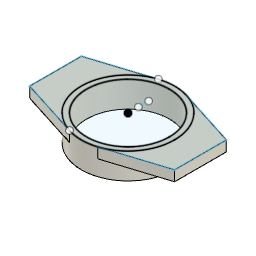
無題 (Autodesk Fusion 360 design; units mm, degrees)
Autodesk Fusion 360 part; units mm, degrees
sketch "スケッチ1" plane through (0, 0, 0) normal (0, 0, 1) x (1, 0, 0)
  circle A0 centre (0, 0) radius 10.5
  circle A1 centre (0, 0) radius 9.5
  circle A2 centre (0, 0) radius 9
  circle A3 centre (0, 0) radius 8
  dimension "d1" = 21
  dimension "d2" = 19
  dimension "d3" = 18
  dimension "d4" = 16
  constraint coincident A0.centre A1.centre
  measures "d1" diameter of A0
  measures "d2" diameter of A1
  measures "d3" diameter of A2
  measures "d4" diameter of A3
extrude "押し出し1" add sketch "スケッチ1" along normal blind 6 contours A0 makes body 1
extrude "押し出し2" add sketch "スケッチ1" along normal blind 6 separate body contours A2 makes body 2
sketch "スケッチ2" plane through (0, 0, 6) normal (0, 0, 1) x (-1, 0, 0)
  circle A0 centre (0, 0) radius 9.5
  circle A1 centre (0, 0) radius 10.5
  line L0 (2, -15) -> (-2, -15)
  line L1 (-2, -15) -> (-8.4577, -6.2223)
  line L2 (2, -15) -> (8.4577, -6.2223)
  line L3 (0, 0) -> (-3.4838, 0)
  line L4 (2, 15) -> (8.4577, 6.2223)
  line L5 (2, 15) -> (-2, 15)
  line L6 (-2, 15) -> (-8.4577, 6.2223)
  constraint horizontal L0
  constraint coincident A1 L1.end
  constraint tangent A1 L1
  constraint coincident A1 L2.end
  constraint tangent A1 L2
  constraint coincident A0.centre A1.centre
  constraint parallel L0 L3
  constraint symmetric L0.start L3 L4.start
  constraint symmetric L0.end L3 L5.end
  constraint symmetric L1.end L3 L6.end
  constraint symmetric L2.end L3 L4.end
extrude "押し出し3" add sketch "スケッチ2" against normal blind 2 contours A1 L4 L5 L6 | A1 L0 L1 L2 bodies 1
sketch "スケッチ3" plane through (0, 0, 6) normal (0, 0, 1) x (-1, 0, 0)
  circle A0 centre (0, 0) radius 8
  circle A1 centre (0, 0) radius 9
  line L0 (-15, -2) -> (-15, 2)
  line L1 (-15, 2) -> (-4.3494, 7.8792)
  line L2 (-15, 0) -> (-12.4057, 0)
  line L3 (-15, -2) -> (-4.3494, -7.8792)
  line L4 (0, 0) -> (0, -2)
  line L5 (15, -2) -> (4.3494, -7.8792)
  line L6 (15, -2) -> (15, 2)
  line L7 (15, 2) -> (4.3494, 7.8792)
  constraint vertical L0
  constraint coincident A1 L1.end
  constraint tangent A1 L1
  constraint midpoint L0 L2.start
  constraint perpendicular L0 L2
  constraint symmetric L0.end L2 L0.start
  constraint symmetric L1.end L2 L3.end
  constraint coincident A0.centre A1.centre
  constraint vertical L4
  constraint symmetric L0.start L4 L5.start
  constraint symmetric L0.end L4 L6.end
  constraint symmetric L1.end L4 L7.end
  constraint symmetric L3.end L4 L5.end
extrude "押し出し4" add sketch "スケッチ3" along normal blind 2 separate body makes body 3
combine "結合1" operation add target body 3 tool bodies 2
sketch "スケッチ1 (2)" plane through (0, 0, 0) normal (0, 0, 1) x (1, 0, 0) in component "Component'"
  circle A0 centre (0, 0) radius 11.25
  circle A1 centre (0, 0) radius 9.75
  line L0 (-2.095, 15.0718) -> (2.1708, 15.0718)
  line L1 (2.1708, 15.0718) -> (8.6891, 7.1458)
  line L2 (-2.095, 15.0718) -> (-8.6482, 7.1952)
  line L3 (-5.0595, -20.013) -> (5.0595, -20.013)
  line L4 (5.0595, -20.013) -> (10.6475, -3.6322)
  line L5 (-5.0595, -20.013) -> (-10.6475, -3.6322)
  dimension "d13" = 22.5
  dimension "d14" = 19.5
  constraint coincident A0.centre A1.centre
  constraint concentric A0 A1
  constraint horizontal L0
  constraint coincident A0 L1.end
  constraint tangent A0 L1
  constraint coincident A0 L2.end
  constraint tangent A0 L2
  constraint horizontal L3
  constraint coincident A0 L4.end
  constraint tangent A0 L4
  constraint coincident A0 L5.end
  constraint tangent A0 L5
  measures "d13" diameter of A0
  measures "d14" diameter of A1
extrude "押し出し1'" add sketch "スケッチ1 (2)" against normal blind 2 separate body makes body 4 in component "Component'"
extrude "押し出し2'" add sketch "スケッチ1 (2)" against normal blind 5 contours A0 bodies 4 in component "Component'"
sketch "スケッチ2 (2)" plane through (0, 0, 0) normal (0, 0, 1) x (1, 0, 0) in component "Component'"
  circle A0 centre (0, 0) radius 9
  circle A1 centre (0, 0) radius 8
  line L0 (14, 5) -> (14, -5)
  line L1 (14, -5) -> (2.722, -8.5785)
  line L2 (14, 5) -> (2.722, 8.5785)
  line L3 (0, 2) -> (0, 4)
  line L4 (-14, 5) -> (-14, -5)
  line L5 (-14, 5) -> (-2.722, 8.5785)
  line L6 (-14, -5) -> (-2.722, -8.5785)
  dimension "d19" = 18
  dimension "d20" = 16
  constraint coincident A0.centre A1.centre
  constraint vertical L0
  constraint coincident A0 L1.end
  constraint tangent A0 L1
  constraint coincident A0 L2.end
  constraint tangent A0 L2
  constraint vertical L3
  constraint symmetric L0.start L3 L4.start
  constraint symmetric L0.end L3 L4.end
  constraint symmetric L1.end L3 L6.end
  constraint symmetric L2.end L3 L5.end
  measures "d19" diameter of A0
  measures "d20" diameter of A1
extrude "押し出し3'" add sketch "スケッチ2 (2)" against normal blind 5 separate body contours A0 makes body 5 in component "Component'"
extrude "押し出し4'" add sketch "スケッチ2 (2)" against normal blind 2 contours A0 L0 L1 L2 | A0 L4 L5 L6 bodies 5 in component "Component'"
component "Component'" placed x (1, 0, 0) y (0, 1, 0) z (0, 0, 1) at (0, 0, 0)
hidden bodies 1 3 4
named bodies: "Out", "Out2", "In2"
